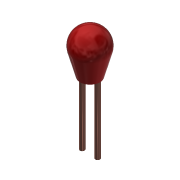
# Autodesk Inventor part: Thermister
Saved by Autodesk Inventor 2017 (Build 210142000, 142)
## iProperties
Created: 2016-12-16
Part Number: Thermister
Material: Generic
Document SubType Name: Modeling
Designer: ge937963
Density: 1 g/cm^3
Appearance: Smooth - Red
Author: ge937963
Autodesk Inventor part; units mm, degrees
ref_plane "YZ Plane" through (0, 0, 0) normal (1, 0, 0) x (0, 1, 0)
ref_plane "XZ Plane" through (0, 0, 0) normal (0, 1, 0) x (-1, 0, 0)
ref_plane "XY Plane" through (0, 0, 0) normal (0, 0, 1) x (1, 0, 0)
sketch "Sketch1" plane through (0, 0, 0) normal (1, 0, 0) x (0, 1, 0)
  arc A0 (0.6188, -0.6126) -> (1.421, 0) centre (0.786, 0) ccw
  line L0 (-0.23, 0) -> (-0.23, -0.381)
  line L1 (-0.23, -0.381) -> (0.6188, -0.6126)
  line L2 (-0.23, 0) -> (1.421, 0)
  line L3 (1.421, 0) -> (1.421, -0.0409)
  point P0 (0, 0)
  dimension "d0" = 0.381
  dimension "d1" = 1.651
  dimension "d2" = 0.635
  constraints: 8 end point, 2 point on circle, 2 tangent, 2 vertical, 1 centre point, 1 horizontal alignment, 1 perpendicular
  measures "d0" distance of L0.start L0.end
  measures "d1" distance from line of L2.end L0
  measures "d2" distance edge to line of A0 L2
revolve "Revolution1" add sketch "Sketch1" angle 360 about axis through (0, -0.23, 0) along (0, 1, 0)
sketch "Sketch2" plane through (0, -0.23, 0) normal (0, -1, 0) x (1, 0, 0)
  circle A0 centre (-0.293, 0) radius 0.0889
  circle A1 centre (0.2912, 0) radius 0.0889
  point P0 (0, 0)
  dimension "d4" = 0.1778
  dimension "d5" = 0.762
  constraints: 2 centre point, 1 equal radius
  measures "d4" diameter of A1
extrude "Extrusion1" add sketch "Sketch2" along normal blind 2.54
body "Solid1"
